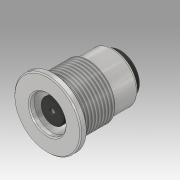
# Autodesk Inventor part: barrel_plug
Saved by Autodesk Inventor 2019.3 (Build 233278000, 278)
## iProperties
Created: 2019-05-29
Part Number: barrel_plug
Material: Generic
Document SubType Name: Modeling
Designer: Dave
Density: 1 g/cm^3
Appearance: Default
Author: Dave
Autodesk Inventor part; units mm, degrees
ref_plane "YZ Plane" through (0, 0, 0) normal (1, 0, 0) x (0, 1, 0)
ref_plane "XZ Plane" through (0, 0, 0) normal (0, 1, 0) x (-1, 0, 0)
ref_plane "XY Plane" through (0, 0, 0) normal (0, 0, 1) x (1, 0, 0)
sketch "Sketch1" plane through (0, 0, 0) normal (0, 0, 1) x (1, 0, 0)
  circle A0 centre (0, 0) radius 7.5
  dimension "d0" = 15
  constraints: 1 centre point, 1 coincident
  measures "d0" diameter of A0
extrude "Extrusion1" add sketch "Sketch1" along normal blind 1.5
sketch "Sketch2" plane through (0, 0, 0) normal (0, 0, -1) x (-1, 0, 0)
  circle A0 centre (0, 0) radius 6
  dimension "d3" = 12
  constraints: 1 centre point, 1 coincident
  measures "d3" diameter of A0
extrude "Extrusion2" add sketch "Sketch2" along normal blind 1.1
sketch "Sketch3" plane through (0, 0, -1.1) normal (0, 0, -1) x (-1, 0, 0)
  circle A0 centre (0, 0) radius 5.995
  dimension "d6" = 11.99
  constraints: 1 centre point, 1 coincident
  measures "d6" diameter of A0
extrude "Extrusion3" add sketch "Sketch3" along normal blind 6.6
sketch "Sketch4" plane through (0, 0, -7.7) normal (0, 0, -1) x (-1, 0, 0)
  circle A0 centre (0, 0) radius 5.5
  dimension "d9" = 11
  constraints: 1 centre point, 1 coincident
  measures "d9" diameter of A0
extrude "Extrusion4" add sketch "Sketch4" along normal blind 5.8
sketch "Sketch5" plane through (0, 0, -13.5) normal (0, 0, -1) x (-1, 0, 0)
  circle A0 centre (0, 0) radius 4.4
  dimension "d12" = 8.8
  constraints: 1 centre point, 1 coincident
  measures "d12" diameter of A0
extrude "Extrusion5" add sketch "Sketch5" along normal blind 1.5
sketch "Sketch6" plane through (0, 0, 1.5) normal (0, 0, 1) x (1, 0, 0)
  circle A0 centre (0, 0) radius 4
  dimension "d15" = 8
  constraints: 1 centre point, 1 coincident
  measures "d15" diameter of A0
extrude "Extrusion6" cut sketch "Sketch6" against normal blind 9.2
sketch "Sketch7" plane through (0, 0, -7.7) normal (0, 0, 1) x (1, 0, 0)
  circle A0 centre (0, 0) radius 4.5
  dimension "d18" = 9
  constraints: 1 centre point, 1 coincident
  measures "d18" diameter of A0
extrude "Extrusion7" cut sketch "Sketch7" along normal blind 8.1
sketch "Sketch8" plane through (0, 0, -7.7) normal (0, 0, 1) x (1, 0, 0)
  circle A0 centre (0, 0) radius 3.5
  dimension "d21" = 7
  constraints: 1 centre point, 1 coincident
  measures "d21" diameter of A0
extrude "Extrusion8" cut sketch "Sketch8" against normal blind 4
sketch "Sketch9" plane through (0, 0, -11.7) normal (0, 0, 1) x (1, 0, 0)
  circle A0 centre (0, 0) radius 2.7
  dimension "d24" = 5.4
  constraints: 1 centre point, 1 coincident
  measures "d24" diameter of A0
extrude "Extrusion9" add sketch "Sketch9" along normal blind 12.1
sketch "Sketch10" plane through (0, 0, 0.4) normal (0, 0, 1) x (1, 0, 0)
  circle A0 centre (0, 0) radius 0.5
  dimension "d27" = 1
  constraints: 1 centre point, 1 coincident
  measures "d27" diameter of A0
extrude "Extrusion10" cut sketch "Sketch10" against normal blind 12.1
sketch "Sketch12" plane through (0, 0, 0) normal (1, 0, 0) x (0, 1, 0)
  line L0 (3.6, -1.4) -> (2.4, -1.4)
  line L1 (2.4, -1.4) -> (2.4, -0.7)
  line L2 (2.4, -0.7) -> (1.6, -0.7)
  line L3 (-1.6, -0.7) -> (-2.4, -0.7)
  line L4 (-2.4, -0.7) -> (-2.4, -1.4)
  line L5 (-2.4, -1.4) -> (-3.6, -1.4)
  line L6 (2.7, 0.4) -> (-2.7, 0.4) projected
  line L7 (3.6, -1.4) -> (3.6, -7.2)
  line L8 (3.6, -7.2) -> (3.1, -7.2)
  line L9 (3.1, -7.2) -> (3.1, -11.7)
  line L10 (3.1, -11.7) -> (1.6, -11.7)
  line L11 (1.6, -11.7) -> (1.6, -0.7)
  line L12 (-3.6, -1.4) -> (-3.6, -7.2)
  line L13 (-3.6, -7.2) -> (-3.1, -7.2)
  line L14 (-3.1, -7.2) -> (-3.1, -11.7)
  line L15 (-1.6, -0.7) -> (-1.6, -11.7)
  line L16 (-1.6, -11.7) -> (-3.1, -11.7)
  line L17 (-0.5, -11.7) -> (0.5, -11.7) projected
  point P0 (0, 0)
  dimension "d38" = 1.1
  dimension "d39" = 0.3
  dimension "d40" = 1.8
  dimension "d48" = 0.3
  dimension "d49" = 1.6
  dimension "d50" = 1.6
  dimension "d51" = 0.5
  dimension "d52" = 4.5
  dimension "d53" = 2
  constraints: 32 end point, 9 perpendicular, 7 point on line, 4 collinear, 2 vertical, 1 parallel
  measures "d38" distance between parallel lines of L2 L6
  measures "d39" distance from line of L6.start L1
  measures "d40" distance between parallel lines of L0 L6
  measures "d48" distance from line of L6.end L4
  measures "d49" distance from line of point (0, 0) L11
  measures "d50" distance from line of L15 point (0, 0)
  measures "d51" distance of L7.end L8.end
  measures "d52" distance of L8.end L9.end
  measures "d53" distance between parallel lines of L15 L12
extrude "Extrusion12" cut sketch "Sketch12" along normal blind 1.2 and the other way blind 1.2
sketch "Sketch13" plane through (0, 0, 0) normal (1, 0, 0) x (0, 1, 0)
  line L0 (1.8233, -1.2) -> (1.6, -1.3124)
  line L1 (1.6, -1.3124) -> (2.6, -3.3)
  line L2 (2.6, -3.3) -> (1.6, -9.6805)
  line L3 (1.6, -9.6805) -> (1.6, -11.7)
  line L4 (1.6, -11.7) -> (1.85, -11.7)
  line L5 (1.85, -11.7) -> (1.85, -9.7)
  line L6 (1.85, -9.7) -> (2.8594, -3.2594)
  line L7 (2.8594, -3.2594) -> (1.8233, -1.2)
  line L8 (1.6, -11.7) -> (1.6, -0.7) projected
  line L9 (2.4187, -11.7) -> (1.6, -11.7) projected
  line L10 (1.6, -0.7) -> (2.4, -0.7) projected
  line L11 (0, 0) -> (0, -11.7) construction
  line L12 (-1.8233, -1.2) -> (-1.6, -1.3124)
  line L13 (-1.6, -1.3124) -> (-2.6, -3.3)
  line L14 (-2.6, -3.3) -> (-1.6, -9.6805)
  line L15 (-1.6, -9.6805) -> (-1.6, -11.7)
  line L16 (-1.6, -11.7) -> (-1.85, -11.7)
  line L17 (-1.85, -11.7) -> (-1.85, -9.7)
  line L18 (-1.85, -9.7) -> (-2.8594, -3.2594)
  line L19 (-2.8594, -3.2594) -> (-1.8233, -1.2)
  line L20 (-1.6, -11.7) -> (-1.6, -0.7)
  line L21 (-2.4187, -11.7) -> (-1.6, -11.7)
  line L22 (-1.6, -0.7) -> (-2.4, -0.7)
  dimension "d58" = 0.25
  dimension "d59" = 0.25
  dimension "d60" = 0.25
  dimension "d61" = 0.25
  dimension "d62" = 2.6
  dimension "d63" = 1
  dimension "d64" = 2
  dimension "d65" = 0.5
  dimension "d66" = 0
  constraints: 40 end point, 12 symmetric about line, 2 collinear, 2 parallel, 2 perpendicular, 2 point on line, 2 vertical
  measures "d58" distance between parallel lines of L1 L7
  measures "d59" distance of L3.end L4.end
  measures "d60" distance between parallel lines of L2 L6
  measures "d61" distance of L0.start L0.end
  measures "d62" distance from line of L1.end L10
  measures "d63" distance from line of L8 L1.end
  measures "d64" distance of L4.end L5.end
  measures "d65" distance from line of L10 L0.start
  measures "d66" distance from line of L11.end L9
extrude "Extrusion13" add sketch "Sketch13" along normal blind 1.1 and the other way blind 1.1 contours L7 L6 L5 L4 L3 L2 L1 L0 | L12 L13 L14 L15 L16 L17 L18 L19
sketch "Sketch14" plane through (0, 0, 0) normal (1, 0, 0) x (0, 1, 0)
  line L0 (0.77, 0) -> (-0.77, 0)
  line L1 (-0.77, 0) -> (-0.77, -11.7)
  line L2 (-0.77, -11.7) -> (0.77, -11.7)
  line L3 (0.77, -11.7) -> (0.77, 0)
  line L4 (-0.5, -11.7) -> (0.5, -11.7) projected
  point P0 (0, 0)
  point P1 (0, 0)
  dimension "d71" = 1.54
  constraints: 8 end point, 2 coincident, 2 parallel, 1 collinear, 1 horizontal, 1 midpoint, 1 perpendicular
  measures "d71" distance between parallel lines of L1 L3
extrude "Extrusion14" cut sketch "Sketch14" against normal blind 1.2 and the other way blind 1.2
sketch "Sketch15" plane through (0, 0, 0) normal (1, 0, 0) x (0, 1, 0)
  line L0 (0.52, 0) -> (0.52, -1.05)
  line L1 (0.52, -1.05) -> (0.25, -2.2)
  line L2 (0.25, -2.2) -> (0.52, -9.6)
  line L3 (0.52, -9.6) -> (0.52, -11.7)
  line L4 (0.52, -11.7) -> (0.77, -11.7)
  line L5 (0.77, -11.7) -> (0.77, -9.5954)
  line L6 (0.77, -9.5954) -> (0.5011, -2.2244)
  line L7 (0.5011, -2.2244) -> (0.77, -1.079)
  line L8 (0.77, -1.079) -> (0.77, 0)
  line L9 (0.77, 0) -> (0.52, 0)
  line L10 (0.77, -11.7) -> (-0.77, -11.7) projected
  line L11 (0, 0) -> (0, -11.7) construction
  line L12 (-0.52, 0) -> (-0.52, -1.05)
  line L13 (-0.52, -1.05) -> (-0.25, -2.2)
  line L14 (-0.25, -2.2) -> (-0.52, -9.6)
  line L15 (-0.52, -9.6) -> (-0.52, -11.7)
  line L16 (-0.52, -11.7) -> (-0.77, -11.7)
  line L17 (-0.77, -11.7) -> (-0.77, -9.5954)
  line L18 (-0.77, -9.5954) -> (-0.5011, -2.2244)
  line L19 (-0.5011, -2.2244) -> (-0.77, -1.079)
  line L20 (-0.77, -1.079) -> (-0.77, 0)
  line L21 (-0.77, 0) -> (-0.52, 0)
  dimension "d76" = 0.25
  dimension "d77" = 0.25
  dimension "d78" = 0.25
  dimension "d79" = 0.25
  dimension "d80" = 1.05
  dimension "d81" = 2.2
  dimension "d82" = 0.25
  dimension "d83" = 2.1
  constraints: 42 end point, 11 symmetric about line, 3 collinear, 3 parallel, 2 perpendicular, 2 vertical alignment, 1 horizontal, 1 horizontal alignment, 1 midpoint, 1 vertical
  measures "d76" distance between parallel lines of L0 L8
  measures "d77" distance between parallel lines of L1 L7
  measures "d78" distance between parallel lines of L2 L6
  measures "d79" distance between parallel lines of L3 L5
  measures "d80" distance of L0.start L0.end
  measures "d81" distance from line of L1.end L9
  measures "d82" horizontal distance of L11.start L1.end
  measures "d83" distance of L2.end L3.end
extrude "Extrusion15" add sketch "Sketch15" along normal blind 1.1 and the other way blind 1.1
thread "Thread1" size "M12x0.75" class "6g" standard "ANSI Metric M Profile" full length
chamfer "Chamfer1" distance 0.25 angle 45 3 edges at (-7.5, 0, 1.5) (-7.5, 0, 0) (-4, 0, 1.5)
fillet "Fillet1" radius 0.25 2 edges at (-2.7, 0, 0.4) (-0.5, 0, 0.4)
fillet "Fillet2" radius 0.5 1 edges at (5.5, 0, -13.5)
fillet "Fillet3" radius 0.25 1 edges at (4.4, 0, -15)
sketch "Sketch16" plane through (0, 0, -15) normal (0, 0, -1) x (-1, 0, 0)
  line L0 (-1.1, -1.85) -> (1.1, -1.85) projected
  line L1 (1.1, -1.85) -> (-1.1, -1.85) projected
  line L2 (1.1, -0.52) -> (-1.1, -0.52) projected
  line L3 (-1.1, -0.52) -> (1.1, -0.52)
  line L4 (1.1, -0.52) -> (1.1, -0.77)
  line L5 (1.1, -0.77) -> (-1.1, -0.77)
  line L6 (-1.1, -0.77) -> (-1.1, -0.52)
  line L7 (-1.1, -2.6) -> (1.1, -2.6)
  line L8 (1.1, -2.6) -> (1.1, -2.95)
  line L9 (1.1, -2.95) -> (-1.1, -2.95)
  line L10 (-1.1, -2.95) -> (-1.1, -2.6)
  dimension "d99" = 2.2
  dimension "d100" = 2.2
  dimension "d101" = 0.25
  dimension "d102" = 0.35
  dimension "d103" = 0.75
  constraints: 16 end point, 4 parallel, 2 horizontal, 2 perpendicular, 2 point on line
  measures "d99" distance of L4.end L5.end
  measures "d100" distance of L8.end L9.end
  measures "d101" distance of L3.end L4.end
  measures "d102" distance of L7.end L8.end
  measures "d103" distance between parallel lines of L0 L7
extrude "Extrusion16" add sketch "Sketch16" along normal blind 2.7
sketch "Sketch17" plane through (-1.1, -2.95, -15) normal (0, -1, 0) x (1, 0, 0)
  circle A0 centre (1.1, -1.7) radius 0.75
  line L0 (0, 0) -> (2.2, 0) projected
  line L1 (0, 0) -> (0, -2.7) projected
  line L2 (2.2, -2.7) -> (0, -2.7) projected
  line L3 (2.2, 0) -> (2.2, -2.7) projected
  point P0 (1.1, 15)
  point P1 (1.1, -2.7)
  dimension "d106" = 1.5
  dimension "d107" = 1
  constraints: 1 centre point, 1 midpoint, 1 vertical alignment
  measures "d106" diameter of A0
  measures "d107" distance of point (1.1, -2.7) A0.centre
extrude "Extrusion17" cut sketch "Sketch17" against normal through all contours A0
fillet "Fillet4" radius 0.5 4 edges at (1.1, -0.645, -17.7) (1.1, -2.775, -17.7) (-1.1, -0.645, -17.7) (-1.1, -2.775, -17.7)
body "Solid1"
